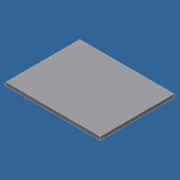
# Autodesk Inventor part: P1704_011_4buttonPCB
Saved by Autodesk Inventor 2019 (Build 230136000, 136)
## iProperties
Created: 2019-05-07
Part Number: P1704_011_4buttonPCB
Project: Nom Projet
Material: .
Description: Nom pièce
Document SubType Name: Modeling
Designer: Joan.MAILLARD
Authority: brut Ø
Density: 0.001 g/cm^3
Appearance: Par défaut
Author: Joan.MAILLARD
Material number: ---
Autodesk Inventor part; units mm, degrees
ref_plane "Plan YZ" through (0, 0, 0) normal (1, 0, 0) x (0, 1, 0)
ref_plane "Plan XZ" through (0, 0, 0) normal (0, 1, 0) x (-1, 0, 0)
ref_plane "Plan XY" through (0, 0, 0) normal (0, 0, 1) x (1, 0, 0)
sketch "Esquisse1" plane through (0, 0, 0) normal (0, 0, 1) x (1, 0, 0)
  line L0 (-26, -20.375) -> (26, -20.375)
  line L1 (26, -20.375) -> (26, 20.375)
  line L2 (26, 20.375) -> (-26, 20.375)
  line L3 (-26, 20.375) -> (-26, -20.375)
  line L4 (-26, -20.375) -> (26, 20.375) construction
  line L5 (26, -20.375) -> (-26, 20.375) construction
  point P0 (0, 0)
  dimension "d0" = 40.75
  dimension "d1" = 52
  constraints: 12 end point, 2 midpoint, 2 parallel, 1 horizontal, 1 perpendicular
  measures "d0" distance of L0.end L1.end
  measures "d1" distance of L1.end L2.end
extrude "Extrusion1" add sketch "Esquisse1" along normal blind 2
